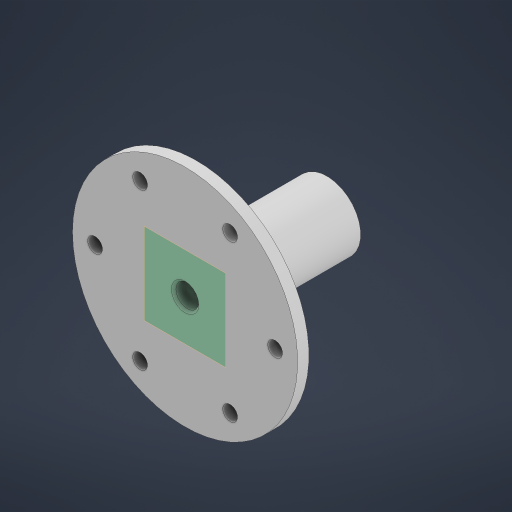
# Autodesk Inventor part: ArmPivot
Saved by Autodesk Inventor 2024.1 (Build 281209000, 209)
## iProperties
Created: 2023-10-16
Part Number: ArmPivot
Material: Generic
Document SubType Name: Modeling
Designer: Brandon
Density: 1 g/cm^3
Appearance: Default
Author: Brandon
Autodesk Inventor part; units mm, degrees
ref_plane "YZ Plane" through (0, 0, 0) normal (1, 0, 0) x (0, 1, 0)
ref_plane "XZ Plane" through (0, 0, 0) normal (0, 1, 0) x (-1, 0, 0)
ref_plane "XY Plane" through (0, 0, 0) normal (0, 0, 1) x (1, 0, 0)
sketch "Sketch1" plane through (0, 0, 0) normal (0, 0, 1) x (1, 0, 0)
  circle A0 centre (4, 0) radius 4 projected
  circle A1 centre (4, 0) radius 3.175 projected
  circle A2 centre (4, 0) radius 3.9492
  circle A3 centre (4, 0) radius 3.2512
  point P0 (0, 0)
  dimension "d0" = 0.0508
  dimension "d1" = 0.0762
  constraints: 2 centre point, 1 horizontal alignment
  measures "d1" radial gap between concentric circles of A1 A3
extrude "Extrusion1" add sketch "Sketch1" along normal blind 15 and the other way blind 57.0076 contours A2
ref_plane "Work Plane1" through (-7, 0, -17.0076) normal (0, 0, -1) x (-1, 0, 0)
sketch "Sketch2" plane through (-7, 0, -17.0076) normal (0, 0, -1) x (-1, 0, 0)
  circle A0 centre (-11, 0) radius 3.9492 projected
  line L0 (-11, 0) -> (126.5, 0)
  line L1 (-11, 0) -> (-561, 0)
  circle A1 centre (-561, 0) radius 12.7
  circle A2 centre (-11, 0) radius 31.75
  line L2 (35.9, 0) -> (-573.7, 0)
  circle A3 centre (-36.4, 0) radius 2.1
  circle A4 centre (-23.7, -21.997) radius 2.1
  circle A5 centre (1.7, -21.997) radius 2.1
  circle A6 centre (14.4, 0) radius 2.1
  circle A7 centre (1.7, 21.997) radius 2.1
  circle A8 centre (-23.7, 21.997) radius 2.1
  line L3 (1.7, -12.7) -> (-23.7, -12.7)
  line L4 (-23.7, -12.7) -> (-23.7, 12.7)
  line L5 (-23.7, 12.7) -> (1.7, 12.7)
  line L6 (1.7, 12.7) -> (1.7, -12.7)
  line L7 (1.7, -12.7) -> (-23.7, 12.7) construction
  line L8 (-23.7, -12.7) -> (1.7, 12.7) construction
  circle A9 centre (-11, 0) radius 9.525
  point P0 (-7, 0)
  dimension "d8" = 25.4
  dimension "d6" = 137.5
  dimension "d7" = 550
  dimension "d9" = 63.5
  dimension "d10" = 609.6
  dimension "d11" = 4.2
  dimension "d12" = 25.4
  dimension "d15" = 360
  dimension "d17" = 25.4
  dimension "d18" = 25.4
  dimension "d19" = 19.05
  constraints: 18 end point, 8 centre point, 4 horizontal, 3 coincident, 2 midpoint, 2 parallel, 2 point on line, 1 horizontal alignment, 1 perpendicular, 15 other
  measures "d6" distance of L0.start L0.end
  measures "d7" distance of L0.start L1.end
  measures "d9" diameter of A2
  measures "d10" distance of L2.start L2.end
  measures "d11" diameter of A3
  measures "d12" distance of L0.start A3.centre
  measures "d17" distance of L4.end L5.end
  measures "d18" distance of L3.end L4.end
  measures "d19" diameter of A9
extrude "Extrusion2" add sketch "Sketch2" along normal blind 40 contours L0 L1 A0 | L0 A9 L1 A0 | A0 L1 L0 | A0 L1 A9 L0
extrude "Extrusion3" add sketch "Sketch2" along normal blind 10.16 contours L0 L1 A0 | L0 A9 L1 A0 | A0 L1 L0 | A0 L1 A9 L0 | A9 L1 L4 L5 L6 L0 | L0 L6 L3 L4 L1 A9
extrude "Extrusion4" add sketch "Sketch2" along normal blind 3.175 contours L6 L5 L4 L1 A3 A2 L0 A6 | L0 A6 A2 L1 A3 L4 L3 L6
sketch "Sketch3" plane through (4, 0, 15) normal (0, 0, 1) x (1, 0, 0)
  line L0 (8.0047, -6.9197) -> (-11.6012, -6.9197)
  line L1 (-11.6012, -6.9197) -> (-11.6012, 5.9412)
  line L2 (-11.6012, 5.9412) -> (8.0047, 5.9412)
  line L3 (8.0047, 5.9412) -> (8.0047, -6.9197)
  point P0 (-4, 0)
  constraints: 8 end point, 2 parallel, 1 horizontal, 1 perpendicular
extrude "Extrusion5" cut sketch "Sketch3" against normal blind 32.0076
sketch "Sketch4" plane through (4, 0, -17.0076) normal (0, 0, 1) x (1, 0, 0)
  circle A0 centre (0, 0) radius 3.175 projected
  circle A1 centre (0, 0) radius 3.2258
  point P0 (-4, 0)
  dimension "d31" = 0.0508
  constraints: 1 centre point
  measures "d31" radial gap between concentric circles of A0 A1
extrude "Extrusion6" cut sketch "Sketch4" against normal blind 40 contours A0 | A1
chamfer "Chamfer2" distance 0.635 angle 45 2 edges at (0.7742, 0, -17.0076) (0.7742, 0, -57.0076)
body "Solid1"
